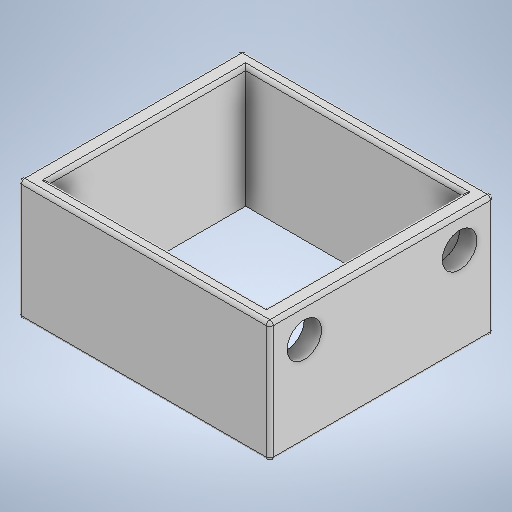
# Autodesk Inventor part: Part185
Saved by Autodesk Inventor 2025 (Build 290162000, 162)
## iProperties
Created: 2024-07-26
Part Number: Part185
Material: Generic
Document SubType Name: Modeling
Designer: Isaac
Density: 1 g/cm^3
Appearance: Default
Author: Isaac
Autodesk Inventor part; units mm, degrees
ref_plane "YZ Plane" through (0, 0, 0) normal (1, 0, 0) x (0, 1, 0)
ref_plane "XZ Plane" through (0, 0, 0) normal (0, 1, 0) x (-1, 0, 0)
ref_plane "XY Plane" through (0, 0, 0) normal (0, 0, 1) x (1, 0, 0)
sketch "Sketch1" plane through (0, 0, 0) normal (0, 0, 1) x (1, 0, 0)
  line L0 (-365, 175) -> (365, 175)
  line L1 (365, 175) -> (365, -175)
  line L2 (365, -175) -> (-365, -175)
  line L3 (-365, -175) -> (-365, 175)
  line L4 (-365, 175) -> (365, -175) construction
  line L5 (365, 175) -> (-365, -175) construction
  point P0 (0, 0)
  dimension "d0" = 730
  dimension "d1" = 350
  constraints: 12 end point, 2 midpoint, 2 parallel, 1 horizontal, 1 perpendicular
  measures "d0" distance of L0.start L0.end
  measures "d1" distance of L2.end L0.start
extrude "Extrusion1" add sketch "Sketch1" along normal blind 650
fillet "Fillet1" radius 10 12 edges at (0, 175, 650) (-365, 175, 325) (0, 175, 0) (365, 175, 325) (365, 0, 650) (365, -175, 325) (365, 0, 0) (0, -175, 650) (-365, 0, 650) (0, -175, 0) (-365, 0, 0) (-365, -175, 325)
sketch "Sketch2" plane through (-355, 175, 10) normal (0, 1, 0) x (1, 0, 0)
  line L0 (670, -30) -> (40, -30)
  line L1 (40, -30) -> (40, -600)
  line L2 (40, -600) -> (670, -600)
  line L3 (670, -600) -> (670, -30)
  line L4 (0, 0) -> (710, 0) projected
  line L5 (710, 0) -> (710, -630) projected
  point P0 (355, 10)
  dimension "d5" = 630
  dimension "d6" = 570
  dimension "d7" = 30
  dimension "d8" = 40
  constraints: 8 end point, 2 parallel, 1 horizontal, 1 perpendicular
  measures "d5" distance of L0.start L0.end
  measures "d6" distance of L2.end L0.start
  measures "d7" distance between parallel lines of L4 L0
  measures "d8" distance between parallel lines of L5 L3
extrude "Extrusion2" cut sketch "Sketch2" against normal blind 350
fillet "Fillet2" radius 10 4 edges at (-315, 175, 325) (0, 175, 40) (0, 175, 610) (315, 175, 325)
sketch "Sketch3" plane through (365, -165, 10) normal (1, 0, 0) x (0, 0, -1)
  circle A0 centre (-540, 250) radius 50
  circle A1 centre (-90, 250) radius 50
  line L0 (-630, 0) -> (-630, 330) projected
  line L1 (0, 330) -> (0, 0) projected
  line L2 (0, 0) -> (-630, 0) projected
  point P0 (10, 165)
  dimension "d12" = 90
  dimension "d13" = 90
  dimension "d14" = 100
  dimension "d15" = 100
  dimension "d16" = 250
  dimension "d17" = 250
  constraints: 2 centre point
  measures "d12" distance from line of L0 A0.centre
  measures "d13" distance from line of L1 A1.centre
  measures "d14" diameter of A0
  measures "d15" diameter of A1
  measures "d16" distance from line of L2 A0.centre
  measures "d17" distance from line of L2 A1.centre
extrude "Extrusion3" cut sketch "Sketch3" against normal blind 350
body "Solid1"
